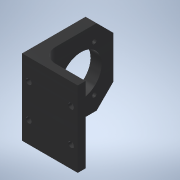
# Autodesk Inventor part: encoder_adapter
Saved by Autodesk Inventor 2021 (Build 250183000, 183)
## iProperties
Created: 2022-04-14
Part Number: encoder_adapter
Material: ABS Plastic
Document SubType Name: Modeling
Designer: 10154704
Density: 1.06 g/cm^3
Appearance: Dark Gray
Mass: 59.4334 g
Surface Area: 175.49 cm^2
Volume: 56.0692 cm^3
Author: 10154704
Autodesk Inventor part; units mm, degrees
note: some values were not read from the file. Chosen so that the rebuilt part matches the saved one: direction of "Bohrung3"; direction of "Bohrung4".
ref_plane "YZ Plane" through (0, 0, 0) normal (1, 0, 0) x (0, 1, 0)
ref_plane "XZ Plane" through (0, 0, 0) normal (0, 1, 0) x (-1, 0, 0)
ref_plane "XY Plane" through (0, 0, 0) normal (0, 0, 1) x (1, 0, 0)
sketch "Skizze1" plane through (0, 0, 0) normal (0, 0, 1) x (1, 0, 0)
  line L0 (0, 0) -> (0, 72)
  line L1 (0, 72) -> (10, 72)
  line L2 (10, 72) -> (10, 7)
  line L3 (10, 7) -> (50, 7)
  line L4 (50, 7) -> (50, 0)
  line L5 (50, 0) -> (0, 0)
  dimension "d0" = 50
  dimension "d27" = 7
  dimension "d43" = 10
  dimension "d45" = 72
  constraints: 12 end point, 5 perpendicular, 1 vertical
  measures "d0" distance of L4.end L0.start
  measures "d27" distance between parallel lines of L5 L3
  measures "d43" distance between parallel lines of L0 L2
  measures "d45" distance between parallel lines of L5 L1
extrude "Extrusion1" add sketch "Skizze1" along normal mid plane 68
sketch "Skizze3" plane through (0, 0, 34) normal (0, -1, 0) x (1, 0, 0)
  line L0 (0, -68) -> (0, 0) projected
  line L1 (50, -68) -> (0, -68) projected
  point P0 (0, -34)
  point P1 (6, -49)
  point P2 (6, -19)
  dimension "d16" = 6
  dimension "d17" = 19
  dimension "d18" = 30
  dimension "d19" = 0
  measures "d16" distance from line of L0 point (6, -49)
  measures "d17" distance from line of L1 point (6, -49)
  measures "d18" distance of point (6, -19) point (6, -49)
  measures "d19" horizontal distance of point (6, -49) point (6, -19)
hole "Bohrung2" at (6, 0, -15) at (6, 0, 15) direction (0, 1, 0) diameter 5 depth 10
sketch "Skizze4" plane through (0, 0, 34) normal (0, -1, 0) x (1, 0, 0)
  circle A0 centre (6, -49) radius 2.5 projected
  circle A1 centre (6, -19) radius 2.5 projected
  point P0 (0, -34)
  point P1 (44, -49)
  point P2 (44, -19)
  dimension "d28" = 38
  dimension "d29" = 38
  dimension "d30" = 0
  dimension "d31" = 0
  measures "d28" distance of point (44, -49) A0.centre
  measures "d29" distance of A1.centre point (44, -19)
  measures "d30" vertical distance of A0.centre point (44, -49)
  measures "d31" vertical distance of A1.centre point (44, -19)
hole "Bohrung3" at (44, 0, -15) at (44, 0, 15) direction (0, 1, 0) diameter 5 end up to surface
sketch "Skizze5" plane through (10, 7, 34) normal (1, 0, 0) x (0, 0, -1)
  circle A0 centre (34, 36) radius 18.5
  line L0 (0, 0) -> (68, 0) projected
  point P0 (34, -7)
  dimension "d42" = 37
  dimension "d46" = 36
  dimension "d47" = 0
  constraints: 1 centre point
  measures "d42" diameter of A0
  measures "d46" distance from line of L0 A0.centre
  measures "d47" horizontal distance of point (34, -7) A0.centre
extrude "Extrusion2" cut sketch "Skizze5" against normal up to surface (10 mm away)
sketch "Skizze8" plane through (20, 7, 34) normal (0, 1, 0) x (1, 0, 0)
  circle A0 centre (24, 19) radius 2.5 projected
  circle A1 centre (24, 49) radius 2.5 projected
  line L0 (28, 21.3094) -> (28, 16.6906)
  line L1 (28, 16.6906) -> (24, 14.3812)
  line L2 (24, 14.3812) -> (20, 16.6906)
  line L3 (20, 16.6906) -> (20, 21.3094)
  line L4 (20, 21.3094) -> (24, 23.6188)
  line L5 (24, 23.6188) -> (28, 21.3094)
  line L6 (24, 44.3812) -> (20, 46.6906)
  line L7 (20, 46.6906) -> (20, 51.3094)
  line L8 (20, 51.3094) -> (24, 53.6188)
  line L9 (24, 53.6188) -> (28, 51.3094)
  line L10 (28, 51.3094) -> (28, 46.6906)
  line L11 (28, 46.6906) -> (24, 44.3812)
  line L12 (30, 0) -> (30, 68) projected
  point P0 (-20, 34)
  point P1 (24, 19)
  point P2 (24, 49)
  dimension "d54" = 8
  dimension "d55" = 8
  constraints: 24 end point, 2 coincident, 2 parallel, 26 other
  measures "d54" distance between parallel lines of L5 L2
  measures "d55" distance between parallel lines of L9 L6
extrude "Extrusion4" cut sketch "Skizze8" against normal blind 4
chamfer "Fase2" distance 15 angle 45 2 edges at (5, 72, -34) (5, 72, 34)
sketch "Skizze9" plane through (0, 0, -34) normal (-1, 0, 0) x (0, 0, 1)
  circle A0 centre (34, 43) radius 18.5 projected
  circle A1 centre (34, 43) radius 18.5 projected
  point P0 (34, 19)
  dimension "d84" = 0
  dimension "d85" = 24
  measures "d84" horizontal distance of A0.centre point (34, 19)
  measures "d85" distance of A0.centre point (34, 19)
hole "Bohrung4" at (0, 19, 0) direction (1, 0, 0) diameter 4 end up to surface counterbore diameter 6 counterbore depth 3
pattern_circular "Runde Anordnung1" count 3 over 360 about axis through (10, 43, 0) along (-1, 0, 0) of "Bohrung4"
fillet "Rundung1" radius 13 1 edges at (10, 7, 0)
sketch "Skizze11" plane through (10, 72, 19) normal (1, 0, 0) x (0, 0, -1)
  circle A0 centre (19, -29) radius 18.5 projected
  circle A1 centre (19, -29) radius 18.5 projected
  circle A2 centre (19, -29) radius 29.5
  point P0 (19, -72)
  dimension "d90" = 59
  constraints: 1 centre point, 1 coincident
  measures "d90" diameter of A2
extrude "Extrusion5" cut sketch "Skizze11" along normal blind 10
equation "\"d29\" = d28"
equation "\"d55\" = d54"
